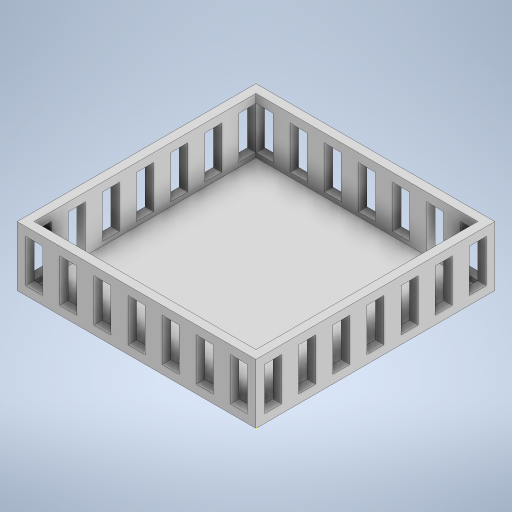
# Autodesk Inventor part: base
Saved by Autodesk Inventor 2024 (Build 280153000, 153)
## iProperties
Created: 2024-01-23
Part Number: base
Material: Generic
Document SubType Name: Modeling
Designer: emosh
Density: 1 g/cm^3
Appearance: Default
Author: emosh
## iProperties of the stored document base_3DPrint.ipt
Created: 2024-01-24
Part Number: base_3DPrint
Material: Generic
Document SubType Name: Modeling
Designer: emosh
Density: 1 g/cm^3
Appearance: Default
Author: emosh
Autodesk Inventor part; units mm, degrees
ref_plane "YZ Plane" through (0, 0, 0) normal (1, 0, 0) x (0, 1, 0)
ref_plane "XZ Plane" through (0, 0, 0) normal (0, 1, 0) x (-1, 0, 0)
ref_plane "XY Plane" through (0, 0, 0) normal (0, 0, 1) x (1, 0, 0)
sketch "Sketch7" plane through (0, 0, 0) normal (0, 1, 0) x (-1, 0, 0)
  line L0 (0, 0) -> (177.8, 0)
  line L1 (177.8, 0) -> (177.8, -177.8)
  line L2 (177.8, -177.8) -> (0, -177.8)
  line L3 (0, -177.8) -> (0, 0)
  line L4 (177.8, 0) -> (171.45, 0)
  line L5 (171.45, 0) -> (171.45, -6.35)
  line L6 (171.45, -6.35) -> (177.8, -6.35)
  line L7 (177.8, -6.35) -> (177.8, 0)
  line L8 (0, -177.8) -> (6.35, -177.8)
  line L9 (6.35, -177.8) -> (6.35, -171.45)
  line L10 (6.35, -171.45) -> (0, -171.45)
  line L11 (0, -171.45) -> (0, -177.8)
  line L12 (171.45, -6.35) -> (6.35, -6.35)
  line L13 (6.35, -6.35) -> (6.35, -171.45)
  line L14 (6.35, -171.45) -> (171.45, -171.45)
  line L15 (171.45, -171.45) -> (171.45, -6.35)
  dimension "d56" = 177.8
  dimension "d57" = 177.8
  dimension "d58" = 6.35
  dimension "d59" = 6.35
  dimension "d60" = 6.35
  dimension "d61" = 6.35
  constraints: 32 end point, 8 parallel, 4 horizontal, 4 perpendicular
  measures "d56" distance of L1.end L2.end
  measures "d57" distance of L0.end L1.end
  measures "d58" distance of L6.end L5.end
  measures "d59" distance of L5.end L4.end
  measures "d60" distance of L10.end L9.end
  measures "d61" distance of L9.end L8.end
extrude "Extrusion7" add sketch "Sketch7" along normal blind 44.45
sketch "Sketch8" plane through (0, 44.45, 0) normal (0, 1, 0) x (1, 0, 0)
  line L0 (-177.8, 177.8) -> (-177.8, 0) projected
  line L1 (-177.8, 177.8) -> (-171.45, 177.8)
  line L2 (-171.45, 177.8) -> (-171.45, 171.45)
  line L3 (-171.45, 171.45) -> (-177.8, 171.45)
  line L4 (-177.8, 171.45) -> (-177.8, 177.8)
  line L5 (-177.8, 0) -> (0, 0) projected
  line L6 (0, 0) -> (-6.35, 0)
  line L7 (-6.35, 0) -> (-6.35, 6.35)
  line L8 (-6.35, 6.35) -> (0, 6.35)
  line L9 (0, 6.35) -> (0, 0)
  line L10 (-6.35, 6.35) -> (-171.45, 6.35)
  line L11 (-171.45, 6.35) -> (-171.45, 171.45)
  line L12 (-171.45, 171.45) -> (-6.35, 171.45)
  line L13 (-6.35, 171.45) -> (-6.35, 6.35)
  dimension "d64" = 6.35
  dimension "d65" = 6.35
  dimension "d66" = 6.35
  dimension "d67" = 6.35
  constraints: 24 end point, 6 parallel, 3 horizontal, 3 perpendicular
  measures "d64" distance of L2.end L3.end
  measures "d65" distance of L1.end L2.end
  measures "d66" distance of L7.end L8.end
  measures "d67" distance of L6.end L7.end
extrude "Extrusion8" cut sketch "Sketch8" against normal blind 41.275 contours L12 L13 L10 L11
sketch "Sketch9" plane through (-177.8, 0, 0) normal (0, 0, 1) x (1, 0, 0)
  point P0 (177.8, 0)
sketch "Sketch12" plane through (-177.8, 0, 0) normal (0, 0, 1) x (1, 0, 0)
  line L0 (177.8, 44.45) -> (0, 44.45) projected
  line L1 (0, 44.45) -> (6.35, 44.45)
  line L2 (6.35, 44.45) -> (6.35, 38.1)
  line L3 (6.35, 38.1) -> (0, 38.1)
  line L4 (0, 38.1) -> (0, 44.45)
  line L5 (177.8, 0) -> (177.8, 44.45) projected
  line L6 (177.8, 0) -> (171.45, 0)
  line L7 (171.45, 0) -> (171.45, 6.35)
  line L8 (171.45, 6.35) -> (177.8, 6.35)
  line L9 (177.8, 6.35) -> (177.8, 0)
  line L10 (171.45, 6.35) -> (6.35, 6.35)
  line L11 (6.35, 6.35) -> (6.35, 38.1)
  line L12 (6.35, 38.1) -> (171.45, 38.1)
  line L13 (171.45, 38.1) -> (171.45, 6.35)
  line L14 (6.35, 38.1) -> (19.05, 38.1)
  line L15 (19.05, 38.1) -> (19.05, 6.35)
  line L16 (19.05, 6.35) -> (6.35, 6.35)
  line L17 (6.35, 6.35) -> (6.35, 38.1)
  line L18 (19.05, 6.35) -> (31.75, 6.35)
  line L19 (31.75, 6.35) -> (31.75, 38.1)
  line L20 (31.75, 38.1) -> (19.05, 38.1)
  line L21 (19.05, 38.1) -> (19.05, 6.35)
  line L22 (31.75, 38.1) -> (44.45, 38.1)
  line L23 (44.45, 38.1) -> (44.45, 6.35)
  line L24 (44.45, 6.35) -> (31.75, 6.35)
  line L25 (31.75, 6.35) -> (31.75, 38.1)
  line L26 (44.45, 6.35) -> (57.15, 6.35)
  line L27 (57.15, 6.35) -> (57.15, 38.1)
  line L28 (57.15, 38.1) -> (44.45, 38.1)
  line L29 (44.45, 38.1) -> (44.45, 6.35)
  line L30 (57.15, 38.1) -> (69.85, 38.1)
  line L31 (69.85, 38.1) -> (69.85, 6.35)
  line L32 (69.85, 6.35) -> (57.15, 6.35)
  line L33 (57.15, 6.35) -> (57.15, 38.1)
  line L34 (69.85, 6.35) -> (82.55, 6.35)
  line L35 (82.55, 6.35) -> (82.55, 38.1)
  line L36 (82.55, 38.1) -> (69.85, 38.1)
  line L37 (69.85, 38.1) -> (69.85, 6.35)
  line L38 (82.55, 38.1) -> (95.25, 38.1)
  line L39 (95.25, 38.1) -> (95.25, 6.35)
  line L40 (95.25, 6.35) -> (82.55, 6.35)
  line L41 (82.55, 6.35) -> (82.55, 38.1)
  line L42 (95.25, 6.35) -> (107.95, 6.35)
  line L43 (107.95, 6.35) -> (107.95, 38.1)
  line L44 (107.95, 38.1) -> (95.25, 38.1)
  line L45 (95.25, 38.1) -> (95.25, 6.35)
  line L46 (107.95, 38.1) -> (120.65, 38.1)
  line L47 (120.65, 38.1) -> (120.65, 6.35)
  line L48 (120.65, 6.35) -> (107.95, 6.35)
  line L49 (107.95, 6.35) -> (107.95, 38.1)
  line L50 (120.65, 6.35) -> (133.35, 6.35)
  line L51 (133.35, 6.35) -> (133.35, 38.1)
  line L52 (133.35, 38.1) -> (120.65, 38.1)
  line L53 (120.65, 38.1) -> (120.65, 6.35)
  line L54 (133.35, 38.1) -> (146.05, 38.1)
  line L55 (146.05, 38.1) -> (146.05, 6.35)
  line L56 (146.05, 6.35) -> (133.35, 6.35)
  line L57 (133.35, 6.35) -> (133.35, 38.1)
  line L58 (146.05, 6.35) -> (158.75, 6.35)
  line L59 (158.75, 6.35) -> (158.75, 38.1)
  line L60 (158.75, 38.1) -> (146.05, 38.1)
  line L61 (146.05, 38.1) -> (146.05, 6.35)
  point P0 (31.75, 6.35)
  point P1 (19.05, 38.1)
  dimension "d109" = 6.35
  dimension "d110" = 6.35
  dimension "d111" = 6.35
  dimension "d112" = 6.35
  dimension "d113" = 12.7
  dimension "d114" = 12.7
  dimension "d115" = 12.7
  dimension "d116" = 12.7
  dimension "d117" = 12.7
  dimension "d118" = 12.7
  dimension "d119" = 12.7
  dimension "d120" = 12.7
  dimension "d121" = 12.7
  dimension "d122" = 12.7
  dimension "d123" = 12.7
  dimension "d124" = 12.7
  constraints: 120 end point, 30 parallel, 15 horizontal, 15 perpendicular, 12 point on line
  measures "d109" distance of L2.end L3.end
  measures "d110" distance of L1.end L2.end
  measures "d111" distance of L7.end L8.end
  measures "d112" distance of L6.end L7.end
  measures "d113" distance of L15.end L16.end
  measures "d114" distance of L20.end L19.end
  measures "d115" distance of L23.end L24.end
  measures "d116" distance of L28.end L27.end
  measures "d117" distance of L31.end L32.end
  measures "d118" distance of L36.end L35.end
  measures "d119" distance of L39.end L40.end
  measures "d120" distance of L44.end L43.end
  measures "d121" distance of L47.end L48.end
  measures "d122" distance of L52.end L51.end
  measures "d123" distance of L55.end L56.end
  measures "d124" distance of L60.end L59.end
extrude "Extrusion11" cut sketch "Sketch12" against normal blind 177.8 contours L12 L15 L10 L11 | L10 L59 L12 L13 | L12 L23 L10 L19 | L10 L51 L12 L55 | L12 L31 L10 L27 | L10 L43 L12 L47 | L12 L39 L10 L35
sketch "Sketch13" plane through (0, 0, 0) normal (1, 0, 0) x (0, 0, -1)
  line L0 (0, 0) -> (0, 44.45) projected
  line L1 (0, 38.1) -> (6.35, 38.1) projected
  line L2 (0, 44.45) -> (6.35, 44.45)
  line L3 (6.35, 44.45) -> (6.35, 38.1)
  line L4 (6.35, 38.1) -> (0, 38.1)
  line L5 (0, 38.1) -> (0, 44.45)
  line L6 (177.8, 0) -> (177.8, 44.45) projected
  line L7 (177.8, 0) -> (171.45, 0)
  line L8 (171.45, 0) -> (171.45, 6.35)
  line L9 (171.45, 6.35) -> (177.8, 6.35)
  line L10 (177.8, 6.35) -> (177.8, 0)
  line L11 (171.45, 6.35) -> (6.35, 6.35)
  line L12 (6.35, 6.35) -> (6.35, 38.1)
  line L13 (6.35, 38.1) -> (171.45, 38.1)
  line L14 (171.45, 38.1) -> (171.45, 6.35)
  line L15 (6.35, 38.1) -> (19.05, 38.1)
  line L16 (19.05, 38.1) -> (19.05, 6.35)
  line L17 (19.05, 6.35) -> (6.35, 6.35)
  line L18 (6.35, 6.35) -> (6.35, 38.1)
  line L19 (19.05, 6.35) -> (31.75, 6.35)
  line L20 (31.75, 6.35) -> (31.75, 38.1)
  line L21 (31.75, 38.1) -> (19.05, 38.1)
  line L22 (19.05, 38.1) -> (19.05, 6.35)
  line L23 (31.75, 38.1) -> (44.45, 38.1)
  line L24 (44.45, 38.1) -> (44.45, 6.35)
  line L25 (44.45, 6.35) -> (31.75, 6.35)
  line L26 (31.75, 6.35) -> (31.75, 38.1)
  line L27 (44.45, 6.35) -> (57.15, 6.35)
  line L28 (57.15, 6.35) -> (57.15, 38.1)
  line L29 (57.15, 38.1) -> (44.45, 38.1)
  line L30 (44.45, 38.1) -> (44.45, 6.35)
  line L31 (57.15, 38.1) -> (69.85, 38.1)
  line L32 (69.85, 38.1) -> (69.85, 6.35)
  line L33 (69.85, 6.35) -> (57.15, 6.35)
  line L34 (57.15, 6.35) -> (57.15, 38.1)
  line L35 (69.85, 6.35) -> (82.55, 6.35)
  line L36 (82.55, 6.35) -> (82.55, 38.1)
  line L37 (82.55, 38.1) -> (69.85, 38.1)
  line L38 (69.85, 38.1) -> (69.85, 6.35)
  line L39 (82.55, 38.1) -> (95.25, 38.1)
  line L40 (95.25, 38.1) -> (95.25, 6.35)
  line L41 (95.25, 6.35) -> (82.55, 6.35)
  line L42 (82.55, 6.35) -> (82.55, 38.1)
  line L43 (95.25, 6.35) -> (107.95, 6.35)
  line L44 (107.95, 6.35) -> (107.95, 38.1)
  line L45 (107.95, 38.1) -> (95.25, 38.1)
  line L46 (95.25, 38.1) -> (95.25, 6.35)
  line L47 (107.95, 38.1) -> (120.65, 38.1)
  line L48 (120.65, 38.1) -> (120.65, 6.35)
  line L49 (120.65, 6.35) -> (107.95, 6.35)
  line L50 (107.95, 6.35) -> (107.95, 38.1)
  line L51 (120.65, 6.35) -> (133.35, 6.35)
  line L52 (133.35, 6.35) -> (133.35, 38.1)
  line L53 (133.35, 38.1) -> (120.65, 38.1)
  line L54 (120.65, 38.1) -> (120.65, 6.35)
  line L55 (133.35, 38.1) -> (146.05, 38.1)
  line L56 (146.05, 38.1) -> (146.05, 6.35)
  line L57 (146.05, 6.35) -> (133.35, 6.35)
  line L58 (133.35, 6.35) -> (133.35, 38.1)
  line L59 (146.05, 6.35) -> (158.75, 6.35)
  line L60 (158.75, 6.35) -> (158.75, 38.1)
  line L61 (158.75, 38.1) -> (146.05, 38.1)
  line L62 (146.05, 38.1) -> (146.05, 6.35)
  dimension "d127" = 6.35
  dimension "d128" = 6.35
  dimension "d129" = 6.35
  dimension "d130" = 6.35
  dimension "d131" = 12.7
  dimension "d132" = 12.7
  dimension "d133" = 12.7
  dimension "d134" = 12.7
  dimension "d135" = 12.7
  dimension "d136" = 12.7
  dimension "d137" = 12.7
  dimension "d138" = 12.7
  dimension "d139" = 12.7
  dimension "d140" = 12.7
  dimension "d141" = 12.7
  dimension "d142" = 12.7
  constraints: 120 end point, 30 parallel, 15 horizontal, 15 perpendicular, 12 point on line
  measures "d127" distance of L1.end L4.end
  measures "d128" distance of L2.end L1.end
  measures "d129" distance of L8.end L9.end
  measures "d130" distance of L7.end L8.end
  measures "d131" distance of L16.end L17.end
  measures "d132" distance of L21.end L20.end
  measures "d133" distance of L24.end L25.end
  measures "d134" distance of L29.end L28.end
  measures "d135" distance of L32.end L33.end
  measures "d136" distance of L37.end L36.end
  measures "d137" distance of L40.end L41.end
  measures "d138" distance of L45.end L44.end
  measures "d139" distance of L48.end L49.end
  measures "d140" distance of L53.end L52.end
  measures "d141" distance of L56.end L57.end
  measures "d142" distance of L61.end L60.end
extrude "Extrusion12" cut sketch "Sketch13" against normal blind 177.8 contours L13 L16 L11 L12 | L13 L24 L11 L20 | L13 L32 L11 L28 | L13 L40 L11 L36 | L13 L48 L11 L44 | L13 L56 L11 L52 | L13 L14 L11 L60
body "Solid2"
